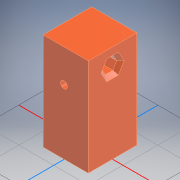
# Autodesk Inventor part: 000.001.001 - Уголок
Saved by Autodesk Inventor 2022 (Build 260153000, 153)
## iProperties
Created: 2022-02-23
Part Number: 000.001.001 - Уголок
Material: Пластик АБС
Document SubType Name: Modeling
Designer: Petrov Ivan
Density: 1.06 g/cm^3
Appearance: Гладкий — белый
Author: Petrov Ivan
Autodesk Inventor part; units mm, degrees
ref_plane "YZ Plane" through (0, 0, 0) normal (1, 0, 0) x (0, 1, 0)
ref_plane "XZ Plane" through (0, 0, 0) normal (0, 1, 0) x (-1, 0, 0)
ref_plane "XY Plane" through (0, 0, 0) normal (0, 0, 1) x (1, 0, 0)
sketch "Эскиз1" plane through (0, 0, 0) normal (0, 1, 0) x (-1, 0, 0)
  line L0 (-14, 14) -> (14, 14)
  line L1 (14, 14) -> (14, -14)
  line L2 (14, -14) -> (-14, -14)
  line L3 (-14, -14) -> (-14, 14)
  line L4 (-14, 14) -> (14, -14) construction
  line L5 (14, 14) -> (-14, -14) construction
  point P0 (0, 0)
  dimension "d0" = 28
  dimension "d1" = 28
  constraints: 12 end point, 2 midpoint, 2 parallel, 1 horizontal, 1 perpendicular
  measures "d0" distance of L1.end L2.end
  measures "d1" distance of L0.end L1.end
extrude "Выдавливание1" add sketch "Эскиз1" along normal blind 56
sketch "Эскиз2" plane through (0, 0, 0) normal (0, -1, 0) x (1, 0, 0)
  circle A0 centre (0, 0) radius 4
  constraints: 1 centre point, 1 coincident
extrude "Выдавливание2" cut sketch "Эскиз2" against normal blind 32
sketch "Эскиз3" plane through (-14, 0, -14) normal (-1, 0, 0) x (0, 0, 1)
  circle A0 centre (14, 46) radius 2
  point P0 (14, 0)
  dimension "d24" = 4
  constraints: 1 centre point
  measures "d24" diameter of A0
extrude "Выдавливание3" cut sketch "Эскиз3" against normal through all
sketch "Эскиз4" plane through (14, 0, 14) normal (1, 0, 0) x (0, 0, -1)
  circle A0 centre (14, 46) radius 2 projected
  line L0 (9.6699, 46) -> (11.8349, 49.75)
  line L1 (11.8349, 49.75) -> (16.1651, 49.75)
  line L2 (16.1651, 49.75) -> (18.3301, 46)
  line L3 (18.3301, 46) -> (16.1651, 42.25)
  line L4 (16.1651, 42.25) -> (11.8349, 42.25)
  line L5 (11.8349, 42.25) -> (9.6699, 46)
  line L6 (0, 56) -> (28, 56) projected
  point P0 (14, 0)
  dimension "d8" = 7.5
  constraints: 12 end point, 1 coincident, 1 parallel, 13 other
  measures "d8" distance between parallel lines of L4 L1
extrude "Выдавливание4" cut sketch "Эскиз4" against normal blind 22
chamfer "Фаска1" distance 2 angle 45 6 edges at (14, 42.25, 0) (14, 44.125, -3.2476) (14, 47.875, -3.2476) (14, 49.75, 0) (14, 47.875, 3.2476) (14, 44.125, 3.2476)
ref_plane "РабПлоскость1" through (0, 22, 0) normal (0, -1, 0) x (1, 0, 0)
sketch "Эскиз5" plane through (0, 22, 0) normal (0, -1, 0) x (1, 0, 0)
  line L0 (0, 8.0829) -> (7, 4.0415)
  line L1 (7, 4.0415) -> (7, -4.0415)
  line L2 (7, -4.0415) -> (0, -8.0829)
  line L3 (0, -8.0829) -> (-7, -4.0415)
  line L4 (-7, -4.0415) -> (-7, 4.0415)
  line L5 (-7, 4.0415) -> (0, 8.0829)
  line L6 (0, 8.0829) -> (-14, 8.0829)
  line L7 (-14, -14) -> (-14, 14) projected
  line L8 (0, -8.0829) -> (-14, -8.0829)
  line L9 (-14, 8.0829) -> (-14, -8.0829)
  point P0 (0, 0)
  point P1 (0, 0)
  dimension "d15" = 14
  constraints: 18 end point, 2 point on line, 1 coincident, 1 collinear, 1 horizontal, 1 parallel, 13 other
  measures "d15" distance between parallel lines of L1 L4
extrude "Выдавливание5" cut sketch "Эскиз5" along normal mid plane 10
move faces "Перенос1" translate (2, 0, 0) faces at (-14, 5.6667, -2.6943)
sketch "Эскиз7" plane through (14, 0, 14) normal (0, 0, 1) x (1, 0, 0)
  line L0 (-10, 32) -> (-18, 32) projected
  line L1 (-2, 42.25) -> (-22, 42.25) projected
  circle A0 centre (-14, 37.125) radius 2
  line L2 (-14, 32) -> (-14, 42.25) construction
  point P0 (-14, 0)
  dimension "d28" = 4
  constraints: 2 end point, 2 midpoint, 1 centre point, 1 coincident, 1 perpendicular, 1 point on line
  measures "d28" diameter of A0
extrude "Выдавливание7" cut sketch "Эскиз7" against normal blind 36.5
sketch "Эскиз8" plane through (14, 0, -14) normal (0, 0, -1) x (-1, 0, 0)
  circle A0 centre (14, 37.125) radius 2 projected
  line L0 (18.3301, 37.125) -> (16.1651, 33.375)
  line L1 (16.1651, 33.375) -> (11.8349, 33.375)
  line L2 (11.8349, 33.375) -> (9.6699, 37.125)
  line L3 (9.6699, 37.125) -> (11.8349, 40.875)
  line L4 (11.8349, 40.875) -> (16.1651, 40.875)
  line L5 (16.1651, 40.875) -> (18.3301, 37.125)
  point P0 (14, 0)
  dimension "d31" = 7.5
  constraints: 12 end point, 1 coincident, 13 other
  measures "d31" distance between parallel lines of L4 L1
extrude "Выдавливание8" cut sketch "Эскиз8" against normal blind 22
equation "\"d1\" = d0"
equation "\"d2\" = 2 * d0"
